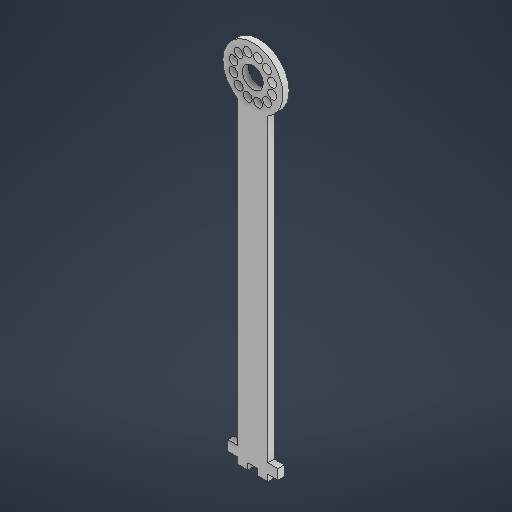
# Autodesk Inventor part: pitahaya1
Saved by Autodesk Inventor 2026.3 (Build 303398000, 398)
## iProperties
Created: 2026-09-15
Part Number: pitahaya1
Material: Generic
Document SubType Name: Modeling
Designer: micha
Density: 1 g/cm^3
Appearance: Default
Author: micha
Autodesk Inventor part; units mm, degrees
ref_plane "YZ Plane" through (0, 0, 0) normal (1, 0, 0) x (0, 1, 0)
ref_plane "XZ Plane" through (0, 0, 0) normal (0, 1, 0) x (-1, 0, 0)
ref_plane "XY Plane" through (0, 0, 0) normal (0, 0, 1) x (1, 0, 0)
sketch "Sketch1" plane through (0, 0, 0) normal (0, 0, 1) x (1, 0, 0)
  line L0 (-6, 60) -> (-6, -60)
  line L1 (-6, -64) -> (-6, -66.5)
  line L2 (-6, -66.5) -> (-2, -66.5)
  line L3 (-2, -66.5) -> (-2, -64)
  line L4 (-2, -64) -> (2, -64)
  line L5 (2, -64) -> (2, -66.5)
  line L6 (2, -66.5) -> (6, -66.5)
  line L7 (6, -66.5) -> (6, -64)
  line L8 (6, -60) -> (6, 60)
  line L9 (0, 63.1461) -> (0, -63.1461) construction
  line L10 (-16.7969, 0) -> (16.7969, 0) construction
  arc A0 (6, 60) -> (-6, 60) centre (0, 70.3923) ccw
  circle A1 centre (-2.0706, 78.1197) radius 1.7678
  line L11 (-2.0706, 90.8634) -> (-2.0706, 65.376) construction
  line L12 (-3.3097, 78.1197) -> (-0.8314, 78.1197) construction
  line L13 (-3.3206, 79.3697) -> (-0.8206, 79.3697) construction
  line L14 (-0.8206, 79.3697) -> (-0.8206, 76.8697) construction
  line L15 (-0.8206, 76.8697) -> (-3.3206, 76.8697) construction
  line L16 (-3.3206, 76.8697) -> (-3.3206, 79.3697) construction
  circle A2 centre (0, 70.3923) radius 8 construction
  line L17 (10, -64) -> (10, -60)
  line L18 (10, -60) -> (6, -60)
  line L19 (-10, -64) -> (-10, -60)
  line L20 (-10, -60) -> (-6, -60)
  line L21 (-10, -64) -> (-6, -64)
  line L22 (6, -64) -> (10, -64)
  line L23 (0, 70.3923) -> (-4.1411, 85.8471) construction
  circle A3 centre (-5.6569, 76.0492) radius 1.7678
  circle A4 centre (-7.7274, 72.4629) radius 1.7678
  circle A5 centre (-7.7274, 68.3218) radius 1.7678
  circle A6 centre (-5.6569, 64.7355) radius 1.7678
  circle A7 centre (-2.0706, 62.6649) radius 1.7678
  circle A8 centre (2.0706, 62.6649) radius 1.7678
  circle A9 centre (5.6569, 64.7355) radius 1.7678
  circle A10 centre (7.7274, 68.3218) radius 1.7678
  circle A11 centre (7.7274, 72.4629) radius 1.7678
  circle A12 centre (5.6569, 76.0492) radius 1.7678
  circle A13 centre (2.0706, 78.1197) radius 1.7678
  line L24 (-4.2764, 70.3923) -> (4.2764, 70.3923) construction
  line L25 (-4, 71.6423) -> (-1.25, 71.6423) construction
  line L26 (-1.25, 71.6423) -> (-1.25, 74.3923) construction
  line L27 (-1.25, 74.3923) -> (1.25, 74.3923) construction
  line L28 (1.25, 74.3923) -> (1.25, 71.6423) construction
  line L29 (1.25, 71.6423) -> (4, 71.6423) construction
  line L30 (4, 71.6423) -> (4, 69.1423) construction
  line L31 (4, 69.1423) -> (1.25, 69.1423) construction
  line L32 (1.25, 69.1423) -> (1.25, 66.3923) construction
  line L33 (1.25, 66.3923) -> (-1.25, 66.3923) construction
  line L34 (-1.25, 66.3923) -> (-1.25, 69.1423) construction
  line L35 (-1.25, 69.1423) -> (-4, 69.1423) construction
  line L36 (-4, 69.1423) -> (-4, 71.6423) construction
  circle A14 centre (0, 70.3923) radius 4.1908
  circle A15 centre (0, 70.3923) radius 6 construction
  point P0 (0, 0)
  point P1 (0, 0)
  point P2 (-5.1993, 77.7567)
  point P3 (-8.1849, 74.1704)
  point P4 (-8.9774, 69.5718)
  point P5 (-7.3644, 65.193)
  point P6 (-3.7781, 62.2074)
  point P7 (0.8206, 61.4149)
  point P8 (5.1993, 63.0279)
  point P9 (8.1849, 66.6142)
  point P10 (8.9774, 71.2129)
  point P11 (7.3644, 75.5916)
  point P12 (3.7781, 78.5772)
  dimension "d9" = 3.5355
  dimension "d10" = 16
  dimension "d0" = 4
  dimension "d2" = 4
  dimension "d7" = 2.5
  dimension "d8" = 2.5
  dimension "d11" = 24
  dimension "d14" = 4
  dimension "d16" = 4
  dimension "d17" = 12
  dimension "d18" = 20
  dimension "d19" = 2.5
  dimension "d20" = 120
  dimension "d21" = 15
  dimension "d24" = 360
  dimension "d28" = 2.5
  dimension "d29" = 2.5
  dimension "d30" = 8
  dimension "d31" = 8
  dimension "d32" = 12
  constraints: 74 end point, 11 perpendicular, 9 point on line, 7 coincident, 7 horizontal, 6 midpoint, 4 horizontal alignment, 4 vertical, 3 vertical alignment, 2 centre point, 2 parallel, 2 point on circle, 1 symmetric about line, 99 other
  measures "d0" distance of L3.end L4.end
  measures "d2" distance of L5.end L6.end
  measures "d7" distance of L15.end L13.start
  measures "d8" distance of L13.start L13.end
  measures "d11" diameter of A0
  measures "d14" distance of L0.end L19.end
  measures "d16" distance of L17.start L17.end
  measures "d17" distance between parallel lines of L8 L0
  measures "d18" distance of L17.start L19.start
  measures "d19" distance of L6.end L7.end
  measures "d20" distance of L0.start L0.end
  measures "d21" angle of L9 L23
  measures "d28" distance of L26.end L27.end
  measures "d29" distance of L35.end L25.start
  measures "d30" distance between parallel lines of L33 L27
  measures "d31" distance between parallel lines of L30 L36
  measures "d32" diameter of A15
extrude "Extrusion1" add sketch "Sketch1" along normal mid plane 2.5
body "Solid1"
